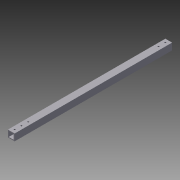
# Autodesk Inventor part: new horizontal kicker thingleft
Saved by Autodesk Inventor 2011 SP1 (Build 150282100, 282)
## iProperties
Created: 2012-01-14
Part Number: new horizontal kicker thingleft
Document SubType Name: Modeling
Designer: Christopher
Density: 1 g/cm^3
Author: Christopher
Autodesk Inventor part; units mm, degrees
ref_plane "YZ Plane" through (0, 0, 0) normal (1, 0, 0) x (0, 1, 0)
ref_plane "XZ Plane" through (0, 0, 0) normal (0, 1, 0) x (-1, 0, 0)
ref_plane "XY Plane" through (0, 0, 0) normal (0, 0, 1) x (1, 0, 0)
sketch "Sketch1" plane through (0, 0, 0) normal (0, 0, 1) x (1, 0, 0)
  line L0 (0, 0) -> (25.4, 0)
  line L1 (25.4, 0) -> (25.4, 25.4)
  line L2 (25.4, 25.4) -> (0, 25.4)
  line L3 (0, 25.4) -> (0, 0)
  line L4 (3.175, 22.225) -> (22.225, 22.225)
  line L5 (22.225, 22.225) -> (22.225, 3.175)
  line L6 (22.225, 3.175) -> (3.175, 3.175)
  line L7 (3.175, 3.175) -> (3.175, 22.225)
  dimension "d0" = 25.4
  dimension "d1" = 25.4
  dimension "d2" = 3.175
  constraints: 16 end point, 4 parallel, 2 perpendicular, 1 horizontal, 3 other
  measures "d0" distance of L1.end L2.end
  measures "d1" distance of L0.end L1.end
  measures "d2" distance between parallel lines of L3 L7
extrude "Extrusion1" add sketch "Sketch1" against normal blind 590.55
sketch "Sketch5" plane through (0, 25.4, 0) normal (0, 1, 0) x (1, 0, 0)
  line L0 (25.4, 590.55) -> (0, 590.55) projected
  line L1 (25.4, 0) -> (0, 0) projected
  point P0 (12.7, 12.7)
  point P1 (12.7, 38.1)
  point P2 (12.7, 63.5)
  point P3 (12.7, 577.85)
  point P4 (12.7, 552.45)
  dimension "d32" = 12.7
  dimension "d33" = 25.4
  dimension "d34" = 12.7
  dimension "d35" = 25.4
  dimension "d36" = 25.4
  measures "d32" distance from line of L0 point (12.7, 577.85)
  measures "d33" distance of point (12.7, 552.45) point (12.7, 577.85)
  measures "d34" distance from line of L1 point (12.7, 12.7)
  measures "d35" distance of point (12.7, 38.1) point (12.7, 12.7)
  measures "d36" distance of point (12.7, 38.1) point (12.7, 63.5)
hole "Hole4" at (12.7, 25.4, -12.7) at (12.7, 25.4, -38.1) at (12.7, 25.4, -63.5) at (12.7, 25.4, -577.85) at (12.7, 25.4, -552.45) direction (0, -1, 0) diameter 5.334 depth 25.4 tip angle 118
body "Solid1"
